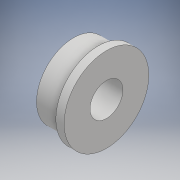
# Autodesk Inventor part: bearing_f684zz
Saved by Autodesk Inventor 2017 (Build 210142000, 142)
## iProperties
Part Number: bearing_f684zz
Material: 一般
Document SubType Name: Modeling
Designer: sktom
Density: 1 g/cm^3
Appearance: 既定
Author: sktom
Autodesk Inventor part; units mm, degrees
ref_plane "YZ Plane" through (0, 0, 0) normal (1, 0, 0) x (0, 1, 0)
ref_plane "XZ Plane" through (0, 0, 0) normal (0, 1, 0) x (-1, 0, 0)
ref_plane "XY Plane" through (0, 0, 0) normal (0, 0, 1) x (1, 0, 0)
sketch "スケッチ1" plane through (0, 0, 0) normal (0, 0, 1) x (1, 0, 0)
  line L0 (0, 2) -> (4, 2)
  line L1 (4, 2) -> (4, 5.15)
  line L2 (4, 5.15) -> (3, 5.15)
  line L3 (3, 5.15) -> (3, 4.5)
  line L4 (3, 4.5) -> (0, 4.5)
  line L5 (0, 4.5) -> (0, 2)
  line L6 (-0.8, 0) -> (4.8, 0) projected
  point P0 (0, 0)
  dimension "d0" = 1
  dimension "d1" = 4
  dimension "d2" = 2
  dimension "d3" = 4.5
  dimension "d4" = 5.15
  constraints: 12 end point, 5 perpendicular, 1 horizontal, 1 vertical alignment
  measures "d0" distance of L1.end L2.end
  measures "d1" distance of L0.start L0.end
  measures "d2" distance from line of point (0, 0) L0
  measures "d3" distance from line of point (0, 0) L4
  measures "d4" distance from line of point (0, 0) L2
revolve "回転1" add sketch "スケッチ1" angle 360 about axis through (-10, 0, 0) along (1, 0, 0)
